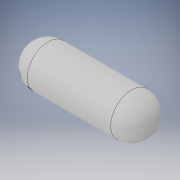
# Autodesk Inventor part: P1704_002_mainDroite
Saved by Autodesk Inventor 2019 (Build 230136000, 136)
## iProperties
Created: 2019-04-29
Part Number: P1704_002_mainDroite
Material: Générique
Document SubType Name: Modeling
Designer: Joan.MAILLARD
Density: 1 g/cm^3
Appearance: Par défaut
Author: Joan.MAILLARD
Autodesk Inventor part; units mm, degrees
ref_plane "YZ Plane" through (0, 0, 0) normal (1, 0, 0) x (0, 1, 0)
sketch "Esquisse1" plane through (0, 0, 0) normal (0, 1, 0) x (-1, 0, 0)
  line L0 (0, 0) -> (-100, 0)
  line L1 (-100, 0) -> (-100, -25)
  line L2 (-100, -25) -> (0, -25)
  line L3 (0, -25) -> (0, 0)
  arc A0 (0, -25) -> (25, 0) centre (0, 0) ccw
  line L4 (25, 0) -> (0, 0)
  line L5 (0, 0) -> (0, -25)
  line L6 (-100, 0) -> (-100, -25)
  arc A1 (-125, 0) -> (-100, -25) centre (-100, 0) ccw
  line L7 (-100, 0) -> (-125, 0)
  dimension "d1" = 25
  dimension "d2" = 100
  constraints: 16 end point, 4 line through centre, 4 point on circle, 3 equal length, 2 centre point, 2 coincident, 2 horizontal, 2 perpendicular, 1 vertical
  measures "d1" distance of L2.end L0.start
  measures "d2" distance of L1.end L2.end
revolve "Révolution1" add sketch "Esquisse1" angle 360 about axis through (0, 0, 0) along (1, 0, 0)
ref_plane "Plan de construction1" through (50, 0, -25) normal (0, 0, 1) x (1, 0, 0)
sketch "Esquisse2" plane through (50, 0, -25) normal (0, 0, 1) x (1, 0, 0)
  arc A0 (-50, 25) -> (-50, -25) centre (-50, 0) ccw projected
  line L0 (-50, 0) -> (-62.5, -21.6506)
  line L1 (-62.5, -21.6506) -> (-84.1506, -9.1506)
  line L2 (-84.1506, -9.1506) -> (-71.6506, 12.5)
  line L3 (-71.6506, 12.5) -> (-50, 0)
  line L4 (-50, 0) -> (-17.1432, 0)
  line L5 (-50, 0) -> (-6.6987, -25)
  line L6 (-6.6987, -25) -> (-19.1987, -46.6506)
  line L7 (-19.1987, -46.6506) -> (-62.5, -21.6506)
  line L8 (-62.5, -21.6506) -> (-50, 0)
  line L9 (-50, -25) -> (-50, 25) construction
  line L10 (-50, -25) -> (100.3384, -25) construction
  dimension "d8" = 120
  constraints: 20 end point, 7 equal length, 2 horizontal, 2 perpendicular, 1 point on circle, 1 point on line
  measures "d8" angle of L0 L4
extrude "Extrusion1" cut sketch "Esquisse2" along normal blind 30
ref_plane "Plan de construction2" through (50, 0, 35) normal (0, 0, -1) x (-1, 0, 0)
sketch "Esquisse3" plane through (50, 0, 35) normal (0, 0, -1) x (-1, 0, 0)
  line L0 (65.2228, -7.3769) -> (52.2324, -14.8769) construction
  circle A0 centre (52.2324, -14.8769) radius 1.7
  circle A1 centre (65.2228, -7.3769) radius 1.7
  line L1 (71.2132, 12.2474) -> (50, 0) construction
  line L2 (71.2132, 12.2474) -> (-7.2, -33.0245) construction
  line L3 (71.2132, 12.2474) -> (83.9867, -9.8769) construction
  dimension "d15" = 3.4
  dimension "d16" = 3.4
  dimension "d23" = 14
  dimension "d24" = 15
  dimension "d25" = 30
  constraints: 6 end point, 2 centre point, 2 coincident, 1 collinear, 1 parallel, 1 perpendicular
  measures "d15" diameter of A1
  measures "d16" diameter of A0
  measures "d23" distance from line of L1 A1.centre
  measures "d24" distance from line of L0.start L3
  measures "d25" distance from line of L0.end L3
extrude "Extrusion2" cut sketch "Esquisse3" along normal blind 30
sketch "Esquisse4" plane through (50, 0, 35) normal (0, 0, -1) x (-1, 0, 0)
  circle A0 centre (65.2228, -7.3769) radius 1.7 projected
  circle A1 centre (65.2228, -7.3769) radius 3.25
  circle A2 centre (52.2324, -14.8769) radius 1.7 projected
  circle A3 centre (52.2324, -14.8769) radius 3.25
  point P0 (50, 0)
  dimension "d19" = 6.5
  dimension "d20" = 6.5
  constraints: 2 centre point, 2 coincident
  measures "d19" diameter of A1
  measures "d20" diameter of A3
extrude "Extrusion3" cut sketch "Esquisse4" along normal blind 20
equation "\"d16\" = d15"
equation "\"d20\" = d19"
